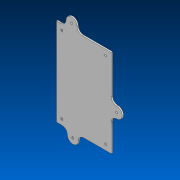
# Autodesk Inventor part: PDP Mount
Saved by Autodesk Inventor 2022 (Build 260153000, 153)
## iProperties
Created: 2022-04-13
Part Number: PDP Mount
Material: Generic
Document SubType Name: Modeling
Designer: score_nygvs6w
Density: 1 g/cm^3
Appearance: Default
Author: score_nygvs6w
Autodesk Inventor part; units mm, degrees
ref_plane "YZ Plane" through (0, 0, 0) normal (1, 0, 0) x (0, 1, 0)
ref_plane "XZ Plane" through (0, 0, 0) normal (0, 1, 0) x (-1, 0, 0)
ref_plane "XY Plane" through (0, 0, 0) normal (0, 0, 1) x (1, 0, 0)
sketch "Sketch1" plane through (0, 0, 0) normal (0, 0, 1) x (1, 0, 0)
  line L0 (50.8, 88.9) -> (-50.8, 88.9) construction
  line L1 (-50.8, 88.9) -> (-50.8, -88.9) construction
  line L2 (-50.8, -88.9) -> (50.8, -88.9) construction
  line L3 (50.8, -88.9) -> (50.8, 88.9) construction
  line L4 (50.8, 88.9) -> (-50.8, -88.9) construction
  line L5 (-50.8, 88.9) -> (50.8, -88.9) construction
  line L6 (-63.5, -101.6) -> (63.5, -101.6)
  line L7 (63.5, -101.6) -> (63.5, 101.6)
  line L8 (63.5, 101.6) -> (-63.5, 101.6)
  line L9 (-63.5, 101.6) -> (-63.5, -101.6)
  line L10 (-63.5, -101.6) -> (63.5, 101.6) construction
  line L11 (63.5, -101.6) -> (-63.5, 101.6) construction
  circle A0 centre (-28.575, 114.3) radius 12.7
  circle A1 centre (76.2, -12.7) radius 12.7
  circle A2 centre (-25.4, -114.3) radius 12.7
  arc A3 (-53.975, 101.6) -> (-41.275, 114.3) centre (-53.975, 114.3) ccw
  arc A4 (-15.875, 114.3) -> (-3.175, 101.6) centre (-3.175, 114.3) ccw
  arc A5 (63.5, 12.7) -> (76.2, 0) centre (76.2, 12.7) ccw
  arc A6 (76.2, -25.4) -> (63.5, -38.1) centre (76.2, -38.1) ccw
  arc A7 (0, -101.6) -> (-12.7, -114.3) centre (0, -114.3) ccw
  arc A8 (-38.1, -114.3) -> (-50.8, -101.6) centre (-50.8, -114.3) ccw
  point P0 (0, 0)
  dimension "d0" = 101.6
  dimension "d1" = 177.8
  dimension "d2" = 12.7
  dimension "d3" = 12.7
  dimension "d13" = 25.4
  dimension "d14" = 127
  dimension "d15" = 104.775
  dimension "d16" = 101.6
  constraints: 24 end point, 18 point on circle, 15 tangent, 9 centre point, 8 equal radius, 7 coincident, 5 midpoint, 5 point on line, 4 parallel, 2 horizontal, 2 perpendicular
  measures "d0" distance of L2.end L1.end
  measures "d1" distance of L1.end L0.end
  measures "d2" distance between parallel lines of L0 L8
  measures "d3" distance between parallel lines of L9 L1
  measures "d13" diameter of A0
  measures "d14" vertical distance of point (76.2, -12.7) point (-28.575, 114.3)
  measures "d15" horizontal distance of point (76.2, -12.7) point (-28.575, 114.3)
  measures "d16" horizontal distance of point (76.2, -12.7) point (-25.4, -114.3)
extrude "Extrusion1" add sketch "Sketch1" along normal blind 3.175
hole "Hole1" at (-50.8, 88.9, 0) at (50.8, 88.9, 0) at (50.8, -88.9, 0) at (-50.8, -88.9, 0) at (-25.4, -114.3, 0) at (76.2, -12.7, 0) at (-28.575, 114.3, 0) direction (0, 0, 1) diameter 4.572 end through all
body "Solid1"
